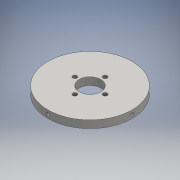
# Autodesk Inventor part: Bottom1
Saved by Autodesk Inventor 2016 (Build 200138000, 138)
## iProperties
Created: 2016-10-25
Part Number: Bottom1
Material: 一般
Document SubType Name: Modeling
Designer: Daisuke
Density: 1 g/cm^3
Appearance: 既定
Author: Daisuke
Autodesk Inventor part; units mm, degrees
sketch "スケッチ1" plane through (0, 0, 0) normal (0, 0, 1) x (1, 0, 0)
  circle A0 centre (0, 0) radius 44.5
  circle A1 centre (0, 0) radius 11.5
  dimension "d0" = 89
  dimension "d1" = 23
  constraints: 2 centre point, 2 coincident
  measures "d0" diameter of A0
  measures "d1" diameter of A1
extrude "押し出し1" add sketch "スケッチ1" along normal blind 8
sketch "スケッチ2" plane through (0, 0, 8) normal (0, 0, 1) x (1, 0, 0)
  line L0 (0, 0) -> (0, 16) construction
  circle A0 centre (0, 16) radius 2.25
  circle A1 centre (-16, 0) radius 2.25
  circle A2 centre (0, -16) radius 2.25
  circle A3 centre (16, 0) radius 2.25
  dimension "d4" = 16
  dimension "d5" = 4.5
  dimension "d8" = 360
  constraints: 4 centre point, 2 end point, 1 coincident, 1 vertical, 9 other
  measures "d4" distance of L0.start L0.end
  measures "d5" diameter of A0
extrude "押し出し2" cut sketch "スケッチ2" against normal blind 8
ref_plane "作業平面1" through (45, 0, 0) normal (1, 0, 0) x (0, 1, 0)
sketch "スケッチ3" plane through (45, 0, 0) normal (1, 0, 0) x (0, 1, 0)
  line L0 (0, 0) -> (0, 4) construction
  circle A0 centre (0, 4) radius 1.5
  dimension "d13" = 4
  dimension "d14" = 3
  constraints: 2 end point, 1 centre point, 1 coincident, 1 vertical
  measures "d13" distance of L0.start L0.end
  measures "d14" diameter of A0
extrude "押し出し3" cut sketch "スケッチ3" against normal blind 5
ref_plane "作業平面2" through (-45, 0, 0) normal (1, 0, 0) x (0, 1, 0)
sketch "スケッチ4" plane through (-45, 0, 0) normal (1, 0, 0) x (0, 1, 0)
  line L0 (0, 0) -> (0, 4) construction
  circle A0 centre (0, 4) radius 1.5
  dimension "d20" = 4
  dimension "d21" = 3
  constraints: 2 end point, 1 centre point, 1 coincident, 1 vertical
  measures "d20" distance of L0.start L0.end
  measures "d21" diameter of A0
extrude "押し出し4" cut sketch "スケッチ4" along normal blind 5
ref_plane "作業平面3" through (0, 45, 0) normal (0, 1, 0) x (-1, 0, 0)
sketch "スケッチ5" plane through (0, 45, 0) normal (0, 1, 0) x (-1, 0, 0)
  line L0 (0, 0) -> (0, 4) construction
  circle A0 centre (0, 4) radius 1.5
  dimension "d25" = 4
  dimension "d26" = 3
  constraints: 2 end point, 1 centre point, 1 coincident, 1 vertical
  measures "d25" distance of L0.start L0.end
  measures "d26" diameter of A0
extrude "押し出し5" cut sketch "スケッチ5" against normal blind 5
ref_plane "作業平面4" through (0, -45, 0) normal (0, 1, 0) x (-1, 0, 0)
sketch "スケッチ6" plane through (0, -45, 0) normal (0, 1, 0) x (-1, 0, 0)
  line L0 (0, 0) -> (0, 4) construction
  circle A0 centre (0, 4) radius 1.5
  dimension "d30" = 4
  dimension "d31" = 3
  constraints: 2 end point, 1 centre point, 1 coincident, 1 vertical
  measures "d30" distance of L0.start L0.end
  measures "d31" diameter of A0
extrude "押し出し6" cut sketch "スケッチ6" along normal blind 5
thread "ねじ2" size "M3x0.5" class "6H" standard "ANSI Metric M Profile" full length
thread "ねじ3" size "M3x0.5" class "6H" standard "ANSI Metric M Profile" full length
thread "ねじ4" size "M3x0.5" class "6H" standard "ANSI Metric M Profile" full length
thread "ねじ5" size "M3x0.5" class "6H" standard "ANSI Metric M Profile" full length
